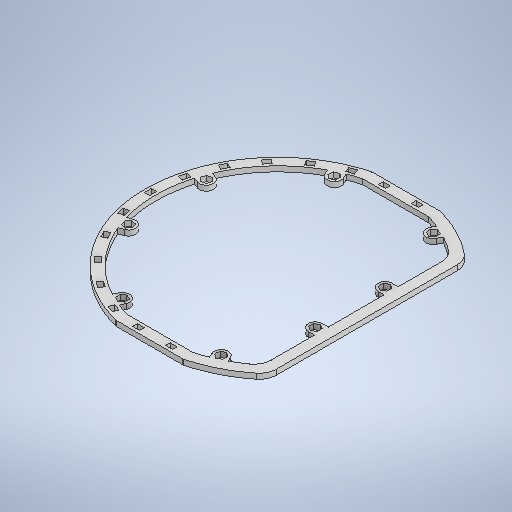
# Autodesk Inventor part: carcasa3.0
Saved by Autodesk Inventor 2025.3 (Build 293356030, 356C)
## iProperties
Created: 2025-08-27
Part Number: carcasa3.0
Material: Generic
Document SubType Name: Modeling
Designer: cdavi
Density: 1 g/cm^3
Appearance: Default
Author: cdavi
Autodesk Inventor part; units mm, degrees
ref_plane "YZ Plane" through (0, 0, 0) normal (1, 0, 0) x (0, 1, 0)
ref_plane "XZ Plane" through (0, 0, 0) normal (0, 1, 0) x (-1, 0, 0)
ref_plane "XY Plane" through (0, 0, 0) normal (0, 0, 1) x (1, 0, 0)
sketch "Sketch1" plane through (0, 0, 0) normal (0, 1, 0) x (-1, 0, 0)
  line L0 (18.2688, 67.5) -> (-18.2688, 67.5)
  line L1 (0, 0) -> (-51, 0) construction
  line L2 (19.0722, 73.5) -> (-19.0722, 73.5)
  line L3 (18.2688, -67.5) -> (-18.5405, -67.5)
  line L4 (19.0722, -73.5) -> (-19.0722, -73.5)
  line L5 (0, 0) -> (0, 73.5) construction
  line L6 (-45, 48.734) -> (-45, -48.734)
  line L7 (-51, 51.7204) -> (-51, -51.7204)
  arc A0 (-40.8333, -56.8563) -> (-18.5405, -67.5) centre (0, 0) ccw
  arc A1 (-47.2121, -59.5568) -> (-19.5877, -73.4324) centre (0, 0) ccw
  arc A2 (19.5877, -73.4324) -> (19.5877, 73.4324) centre (0, 0) ccw
  arc A3 (-19.5877, 73.4324) -> (-47.2121, 59.5568) centre (0, 0) ccw
  arc A4 (18.8061, -67.4265) -> (18.8061, 67.4265) centre (0, 0) ccw
  arc A5 (-18.8061, 67.4265) -> (-40.8333, 56.8563) centre (0, 0) ccw
  arc A6 (-19.5877, -73.4324) -> (-19.0722, -73.5) centre (-19.0722, -71.5) ccw
  arc A7 (19.0722, -73.5) -> (19.5877, -73.4324) centre (19.0722, -71.5) ccw
  arc A8 (18.2688, -67.5) -> (18.8061, -67.4265) centre (18.2688, -65.5) ccw
  arc A9 (18.8061, 67.4265) -> (18.2688, 67.5) centre (18.2688, 65.5) ccw
  arc A10 (19.5877, 73.4324) -> (19.0722, 73.5) centre (19.0722, 71.5) ccw
  arc A11 (-18.2688, 67.5) -> (-18.8061, 67.4265) centre (-18.2688, 65.5) ccw
  arc A12 (-19.0722, 73.5) -> (-19.5877, 73.4324) centre (-19.0722, 71.5) ccw
  arc A13 (-40.8333, 56.8563) -> (-45, 48.734) centre (-35, 48.734) ccw
  arc A14 (-47.2121, 59.5568) -> (-51, 51.7204) centre (-41, 51.7204) ccw
  arc A15 (-51, -51.7204) -> (-47.2121, -59.5568) centre (-41, -51.7204) ccw
  arc A16 (-45, -48.734) -> (-40.8333, -56.8563) centre (-35, -48.734) ccw
  point P0 (-19.3326, 73.5)
  point P1 (18.5405, -67.5)
  point P2 (19.3326, -73.5)
  point P3 (-19.3326, -73.5)
  point P4 (-51, -56.3471)
  point P5 (-45, 53.619)
  point P6 (-45, -53.619)
  point P7 (-51, 56.3471)
  point P8 (19.3326, 73.5)
  point P9 (18.5405, 67.5)
  point P10 (-18.5405, 67.5)
  dimension "d2" = 67.5
  dimension "d4" = 6
  dimension "d6" = 45
  dimension "d7" = 6
  dimension "d8" = 2
  dimension "d9" = 10
  dimension "d10" = 70
  dimension "d11" = 76
  dimension "d12" = 70
  dimension "d13" = 76
  constraints: 45 point on circle, 22 tangent, 17 centre point, 16 end point, 11 point on line, 9 equal radius, 4 symmetric about line, 3 vertical, 2 coincident, 2 horizontal, 2 midpoint, 1 parallel
  measures "d2" distance between parallel lines of L1 L0
  measures "d4" distance between parallel lines of L0 L2
  measures "d6" distance between parallel lines of L6 L5
  measures "d7" distance between parallel lines of L7 L6
  measures "d8" radius of A6
  measures "d9" radius of A13
  measures "d10" radius of A4
  measures "d11" radius of A2
  measures "d12" radius of A0
  measures "d13" radius of A1
extrude "Extrusion1" add sketch "Sketch1" along normal blind 65
sketch "Sketch2" plane through (51, 0, 51.7204) normal (1, 0, 0) x (0, 0, -1)
  line L0 (51.7204, 0) -> (51.7204, 65) construction
  line L1 (100.4544, 65) -> (2.9864, 65) projected
  line L2 (-2.712, 38) -> (17.288, 38)
  line L3 (17.288, 38) -> (17.288, 26)
  line L4 (17.288, 26) -> (-2.712, 26)
  line L5 (-2.712, 26) -> (-2.712, 38)
  line L6 (0, 0) -> (103.4408, 0) projected
  line L7 (-21.712, 0) -> (-21.712, 65) projected
  line L8 (106.1528, 38) -> (86.1528, 38)
  line L9 (86.1528, 38) -> (86.1528, 26)
  line L10 (86.1528, 26) -> (106.1528, 26)
  line L11 (106.1528, 26) -> (106.1528, 38)
  dimension "d16" = 26
  dimension "d17" = 19
  dimension "d18" = 12
  dimension "d19" = 20
  constraints: 18 end point, 4 symmetric about line, 2 parallel, 1 horizontal, 1 midpoint, 1 perpendicular
  measures "d16" distance between parallel lines of L6 L4
  measures "d17" distance between parallel lines of L5 L7
  measures "d18" distance of L2.end L3.end
  measures "d19" distance of L2.start L2.end
extrude "Extrusion2" cut sketch "Sketch2" against normal blind 5
sketch "Sketch3" plane through (51, 0, 51.7204) normal (1, 0, 0) x (0, 0, -1)
  line L0 (3.568, 49.2223) -> (17.7975, 43.9952) construction
  line L1 (2.8909, 47.379) -> (17.1204, 42.1519)
  line L2 (18.4746, 45.8385) -> (4.2452, 51.0656)
  arc A0 (4.2452, 51.0656) -> (2.8909, 47.379) centre (3.568, 49.2223) ccw
  arc A1 (17.1204, 42.1519) -> (18.4746, 45.8385) centre (17.7975, 43.9952) ccw
  arc A2 (44.4296, 11.624) -> (34.6921, 2.9774) centre (43.8866, 2.4292) ccw construction
  arc A3 (44.531, 13.3402) -> (32.9759, 3.0797) centre (43.8866, 2.4292) ccw
  arc A4 (44.3283, 9.9077) -> (36.4083, 2.8751) centre (43.8866, 2.4292) ccw
  arc A5 (44.3283, 9.9077) -> (44.531, 13.3402) centre (44.4296, 11.624) ccw
  arc A6 (32.9759, 3.0797) -> (36.4083, 2.8751) centre (34.6921, 2.9774) ccw
  line L3 (51.7204, 0) -> (51.7204, 65) construction
  line L4 (100.5499, 47.379) -> (86.3204, 42.1519)
  line L5 (84.9662, 45.8385) -> (99.1956, 51.0656)
  arc A7 (100.5499, 47.379) -> (99.1956, 51.0656) centre (99.8728, 49.2223) ccw
  arc A8 (84.9662, 45.8385) -> (86.3204, 42.1519) centre (85.6433, 43.9952) ccw
  point P0 (10.6828, 46.6088)
  constraints: 18 point on circle, 12 end point, 9 centre point, 8 tangent, 6 symmetric about line, 1 midpoint, 1 parallel, 2 other
extrude "Extrusion3" [suppressed]
extrude "Extrusion4" add sketch "Sketch1" along normal blind 3 from surface at 65 separate body contours A9 A4 A8 L3 A0 A16 L6 A13 A5 A11 L0 | A10 A2 A7 L4 A6 A1 A15 L7 A14 A3 A12 L2
sketch "Sketch5" plane through (-19.0722, 68, 73.5) normal (0, 1, 0) x (1, 0, 0)
  circle A0 centre (19.0722, 73.5) radius 8.5
  circle A1 centre (-10.9278, 73.5) radius 2.5
  line L0 (27.1963, 71) -> (36.0722, 71)
  line L1 (36.0722, 71) -> (36.0722, 76)
  line L2 (36.0722, 76) -> (27.1963, 76)
  point P0 (36.0722, 73.5)
  dimension "d26" = 17
  dimension "d27" = 5
  dimension "d31" = 5
  dimension "d32" = 17
  dimension "d47" = 30
  constraints: 6 end point, 2 centre point, 2 horizontal alignment, 2 perpendicular, 2 point on circle, 1 coincident, 1 horizontal, 1 midpoint
  measures "d26" diameter of A0
  measures "d27" diameter of A1
  measures "d31" distance between parallel lines of L2 L0
  measures "d32" distance from line of A0.centre L1
  measures "d47" distance of A0.centre A1.centre
extrude "Extrusion5" cut sketch "Sketch5" against normal through all bodies 2
sketch "Sketch6" plane through (0, 0, 0) normal (0, 1, 0) x (-1, 0, 0)
  circle A0 centre (0, 0) radius 67 construction
  arc A1 (-18.8061, 67.4265) -> (-40.8333, 56.8563) centre (0, 0) ccw projected
  arc A2 (-40.8333, 56.8563) -> (-45, 48.734) centre (-35, 48.734) ccw projected
  line L0 (-45, -48.734) -> (-45, 48.734) projected
  arc A3 (-45, -48.734) -> (-40.8333, -56.8563) centre (-35, -48.734) ccw projected
  arc A4 (-40.8333, -56.8563) -> (-18.5405, -67.5) centre (0, 0) ccw projected
  line L1 (18.2688, -67.5) -> (-18.5405, -67.5) construction
  arc A5 (18.8061, -67.4265) -> (18.8061, 67.4265) centre (0, 0) ccw projected
  line L2 (-18.2688, 67.5) -> (18.2688, 67.5) construction
  line L3 (19.0722, 73.5) -> (-19.0722, 73.5) projected
  arc A6 (-19.5877, 73.4324) -> (-47.2121, 59.5568) centre (0, 0) ccw projected
  arc A7 (-47.2121, 59.5568) -> (-51, 51.7204) centre (-41, 51.7204) ccw projected
  line L4 (-51, 51.7204) -> (-51, -51.7204) projected
  arc A8 (-51, -51.7204) -> (-47.2121, -59.5568) centre (-41, -51.7204) ccw projected
  arc A9 (-47.2121, -59.5568) -> (-19.5877, -73.4324) centre (0, 0) ccw projected
  line L5 (-19.0722, -73.5) -> (19.0722, -73.5) projected
  arc A10 (19.5877, -73.4324) -> (19.5877, 73.4324) centre (0, 0) ccw projected
  arc A11 (-17.9906, 61.4194) -> (-37.3333, 51.9829) centre (0, 0) ccw construction
  arc A12 (-37.3333, 51.9829) -> (-39, 48.734) centre (-35, 48.734) ccw construction
  line L6 (-39, 48.734) -> (-39, -48.734) construction
  arc A13 (-39, -48.734) -> (-37.3333, -51.9829) centre (-35, -48.734) ccw construction
  arc A14 (-37.3333, -51.9829) -> (-17.9906, -61.4194) centre (0, 0) ccw construction
  line L7 (-17.4284, -61.5) -> (17.4284, -61.5) construction
  line L8 (-17.4284, 61.5) -> (17.4284, 61.5) construction
  arc A15 (17.9906, -61.4194) -> (17.9906, 61.4194) centre (0, 0) ccw construction
  arc A16 (-8.124, -2.5) -> (-8.124, 2.5) centre (0, 0) ccw projected
  line L9 (0, 0) -> (63.1919, 22.2662) construction
  line L10 (0, 0) -> (76, 0) construction
  circle A17 centre (63.1919, 22.2662) radius 2.85 construction
  line L11 (0, 0) -> (0, -67) construction
  circle A18 centre (28.3154, 60.7226) radius 2.85 construction
  line L12 (28.3154, 60.7226) -> (0, 0) construction
  circle A19 centre (-41.5, 20) radius 2.85 construction
  circle A20 centre (-28.3154, 60.7226) radius 2.85 construction
  line L13 (-28.3154, 60.7226) -> (0, 0) construction
  arc A21 (-17.4284, 61.5) -> (-17.9906, 61.4194) centre (-17.4284, 59.5) ccw construction
  arc A22 (-17.9906, -61.4194) -> (-17.4284, -61.5) centre (-17.4284, -59.5) ccw construction
  arc A23 (17.4284, -61.5) -> (17.9906, -61.4194) centre (17.4284, -59.5) ccw construction
  arc A24 (17.9906, 61.4194) -> (17.4284, 61.5) centre (17.4284, 59.5) ccw construction
  arc A25 (-19.5877, -73.4324) -> (-19.0722, -73.5) centre (-19.0722, -71.5) ccw projected
  arc A26 (19.0722, -73.5) -> (19.5877, -73.4324) centre (19.0722, -71.5) ccw projected
  arc A27 (19.5877, 73.4324) -> (19.0722, 73.5) centre (19.0722, 71.5) ccw projected
  arc A28 (-19.0722, 73.5) -> (-19.5877, 73.4324) centre (-19.0722, 71.5) ccw projected
  circle A29 centre (63.1919, -22.2662) radius 2.85 construction
  circle A30 centre (28.3154, -60.7226) radius 2.85 construction
  circle A31 centre (-41.5, -20) radius 2.85 construction
  circle A32 centre (-28.3154, -60.7226) radius 2.85 construction
  line L14 (18.8061, 61.1746) -> (18.8061, 67.4265)
  line L15 (-18.8061, 61.1746) -> (-18.8061, 67.4265)
  line L16 (18.8061, 67.4265) -> (-18.8061, 67.4265)
  line L17 (18.8061, -61.1746) -> (18.8061, -67.4265)
  line L18 (-18.8061, -61.1746) -> (-18.8061, -67.4265)
  line L19 (18.8061, -67.4265) -> (-18.8061, -67.4265)
  circle A33 centre (63.1919, 22.2662) radius 4
  circle A34 centre (28.3154, 60.7226) radius 4
  line L20 (60.3905, 22.7899) -> (62.2448, 24.9542)
  line L21 (62.2448, 24.9542) -> (65.0462, 24.4304)
  line L22 (65.0462, 24.4304) -> (65.9934, 21.7424)
  line L23 (65.9934, 21.7424) -> (64.1391, 19.5782)
  line L24 (64.1391, 19.5782) -> (61.3376, 20.1019)
  line L25 (61.3376, 20.1019) -> (60.3905, 22.7899)
  line L26 (25.9808, 59.0879) -> (25.7324, 61.9271)
  line L27 (25.7324, 61.9271) -> (28.067, 63.5618)
  line L28 (28.067, 63.5618) -> (30.65, 62.3573)
  line L29 (30.65, 62.3573) -> (30.8984, 59.5182)
  line L30 (30.8984, 59.5182) -> (28.5638, 57.8835)
  line L31 (28.5638, 57.8835) -> (25.9808, 59.0879)
  circle A35 centre (-41.5, 20) radius 4
  line L32 (-43.9682, 18.575) -> (-43.9682, 21.425)
  line L33 (-43.9682, 21.425) -> (-41.5, 22.85)
  line L34 (-41.5, 22.85) -> (-39.0318, 21.425)
  line L35 (-39.0318, 21.425) -> (-39.0318, 18.575)
  line L36 (-39.0318, 18.575) -> (-41.5, 17.15)
  line L37 (-41.5, 17.15) -> (-43.9682, 18.575)
  line L38 (-41.5, 24) -> (-45, 24)
  line L39 (-41.5, 16) -> (-45, 16)
  circle A36 centre (-28.3154, 60.7226) radius 4
  line L40 (-28.5638, 57.8835) -> (-30.8984, 59.5182)
  line L41 (-30.8984, 59.5182) -> (-30.65, 62.3573)
  line L42 (-30.65, 62.3573) -> (-28.067, 63.5618)
  line L43 (-28.067, 63.5618) -> (-25.7324, 61.9271)
  line L44 (-25.7324, 61.9271) -> (-25.9808, 59.0879)
  line L45 (-25.9808, 59.0879) -> (-28.5638, 57.8835)
  line L46 (-31.8886, 58.9247) -> (-33.2376, 61.6057)
  circle A37 centre (63.1919, -22.2662) radius 4
  circle A38 centre (28.3154, -60.7226) radius 4
  circle A39 centre (-41.5, -20) radius 4
  line L47 (-41.5, -24) -> (-45, -24)
  line L48 (-41.5, -16) -> (-45, -16)
  circle A40 centre (-28.3154, -60.7226) radius 4
  line L49 (-31.8886, -58.9247) -> (-33.2376, -61.6057)
  line L50 (60.3905, -22.7899) -> (62.2448, -24.9542)
  line L51 (62.2448, -24.9542) -> (65.0462, -24.4304)
  line L52 (65.0462, -24.4304) -> (65.9934, -21.7424)
  line L53 (65.9934, -21.7424) -> (64.1391, -19.5782)
  line L54 (64.1391, -19.5782) -> (61.3376, -20.1019)
  line L55 (61.3376, -20.1019) -> (60.3905, -22.7899)
  line L56 (25.9808, -59.0879) -> (25.7324, -61.9271)
  line L57 (25.7324, -61.9271) -> (28.067, -63.5618)
  line L58 (28.067, -63.5618) -> (30.65, -62.3573)
  line L59 (30.65, -62.3573) -> (30.8984, -59.5182)
  line L60 (30.8984, -59.5182) -> (28.5638, -57.8835)
  line L61 (28.5638, -57.8835) -> (25.9808, -59.0879)
  line L62 (-28.5638, -57.8835) -> (-30.8984, -59.5182)
  line L63 (-30.8984, -59.5182) -> (-30.65, -62.3573)
  line L64 (-30.65, -62.3573) -> (-28.067, -63.5618)
  line L65 (-28.067, -63.5618) -> (-25.7324, -61.9271)
  line L66 (-25.7324, -61.9271) -> (-25.9808, -59.0879)
  line L67 (-25.9808, -59.0879) -> (-28.5638, -57.8835)
  line L68 (-43.9682, -18.575) -> (-43.9682, -21.425)
  line L69 (-43.9682, -21.425) -> (-41.5, -22.85)
  line L70 (-41.5, -22.85) -> (-39.0318, -21.425)
  line L71 (-39.0318, -21.425) -> (-39.0318, -18.575)
  line L72 (-39.0318, -18.575) -> (-41.5, -17.15)
  line L73 (-41.5, -17.15) -> (-43.9682, -18.575)
  line L74 (61.7506, 25.9975) -> (64.5502, 27.0789)
  line L75 (64.408, 18.4555) -> (67.2672, 19.368)
  line L76 (31.8886, 58.9247) -> (33.2376, 61.6057)
  line L77 (61.7506, -25.9975) -> (64.5502, -27.0789)
  line L78 (64.408, -18.4555) -> (67.2672, -19.368)
  line L79 (31.8886, -58.9247) -> (33.2376, -61.6057)
  line L80 (-24.6413, 62.3041) -> (-25.828, 65.0609)
  line L81 (24.6413, 62.3041) -> (25.828, 65.0609)
  line L82 (-24.6413, -62.3041) -> (-25.828, -65.0609)
  line L83 (24.6413, -62.3041) -> (25.828, -65.0609)
  point P0 (-17.713, -61.5)
  point P1 (-18.8061, 61.1746)
  point P2 (18.8061, -61.1746)
  point P3 (-18.8061, -61.1746)
  point P4 (28.3154, 60.7226)
  point P5 (28.3154, 60.7226)
  point P6 (-18.8061, -67.4265)
  point P7 (-27.1107, 64.5369)
  point P8 (-27.1107, -64.5369)
  point P9 (27.1107, -64.5369)
  point P10 (27.1107, 64.5369)
  point P11 (-45, 21.9365)
  point P12 (-45, 18.0635)
  point P13 (-32.0117, 62.2515)
  point P14 (32.0117, -62.2515)
  point P15 (66.8707, -20.6956)
  point P16 (65.0736, -25.796)
  point P17 (-32.0117, -62.2515)
  point P18 (-45, -21.9365)
  point P19 (-45, -18.0635)
  point P20 (65.0736, 25.796)
  point P21 (66.8707, 20.6956)
  point P22 (32.0117, 62.2515)
  dimension "d33" = 134
  dimension "d39" = 5.7
  dimension "d34" = 6
  dimension "d35" = 6
  dimension "d36" = 6
  dimension "d37" = 19.41
  dimension "d38" = 25
  dimension "d40" = 20
  dimension "d41" = 3.5
  dimension "d42" = 25
  dimension "d44" = 2
  dimension "d61" = 8
  dimension "d62" = 8
  dimension "d63" = 8
  dimension "d64" = 8
  constraints: 156 end point, 52 symmetric about line, 37 point on circle, 20 centre point, 16 tangent, 10 coincident, 6 perpendicular, 3 equal radius, 3 point on line, 2 parallel, 2 vertical, 93 other
  measures "d34" radial gap between concentric circles of A1 A11
  measures "d35" distance between parallel lines of L2 L8
  measures "d36" radial gap between concentric circles of A5 A15
  measures "d37" angle of L10 L9
  measures "d38" angle of L11 L12
  measures "d40" distance from line of point (-41.5, 20) L10
  measures "d41" distance from line of L0 point (-41.5, 20)
  measures "d42" angle of L11 L13
  measures "d44" radius of A21
  measures "d61" diameter of A33
  measures "d62" diameter of A34
  measures "d63" diameter of A35
  measures "d64" diameter of A36
extrude "Extrusion6" add sketch "Sketch6" against normal blind 3 separate body contours L80 A36 A1 | A36 A1 | A1 A36 | A5 A34 L81 | A36 L46 A1 | A34 A5 | A5 A34 | A5 L76 A34 | A5 A33 L74 | L38 A35 L0 | A33 A5 | A5 A33 | A35 L0 | L0 A35 | A5 L75 A33 | A35 L39 L0 | A5 A37 L78 | L48 A39 L0 | A37 A5 | A5 A37 | A39 L0 | L0 A39 | A5 L77 A37 | A39 L47 L0 | A5 A38 L79 | A38 A5 | A5 A38 | A5 L83 A38 | L49 A40 A4 | A40 A4 | A4 A40 | A40 L82 A4 | A27 A10 A26 L5 A25 A9 A8 L4 A7 A6 A28 L3
sketch "Sketch7" plane through (0, 0, 0) normal (0, 1, 0) x (1, 0, 0)
  line L0 (-43.1612, -69.503) -> (-43.1612, 69.6172)
  line L1 (-23.8326, -59.397) -> (-23.8326, -67.4265) projected
  line L2 (-94.0019, 0.3288) -> (-72.5423, 0.3288)
  line L3 (-72.5423, 0.3288) -> (-72.5423, -7.6712)
  line L4 (-72.5423, 0.3288) -> (-72.5423, 8.3288)
  arc A0 (-19.5877, 73.4324) -> (-19.5877, -73.4324) centre (0, 0) ccw projected
  line L5 (-72.5423, -7.6712) -> (-75.5423, -7.6712)
  line L6 (-75.5423, -7.6712) -> (-75.5423, 8.3288)
  line L7 (-75.5423, 8.3288) -> (-72.5423, 8.3288)
  line L8 (-68.8178, -24.1938) -> (-71.7369, -24.8857)
  line L9 (-71.7369, -24.8857) -> (-75.4267, -9.317)
  line L10 (-70.6627, -16.4095) -> (-68.8178, -24.1938)
  line L11 (-70.6627, -16.4095) -> (-72.5076, -8.6251)
  line L12 (-75.4267, -9.317) -> (-72.5076, -8.6251)
  line L13 (-61.3833, -39.4122) -> (-64.0642, -40.7586)
  line L14 (-64.0642, -40.7586) -> (-71.245, -26.4604)
  line L15 (-64.9737, -32.2631) -> (-61.3833, -39.4122)
  line L16 (-64.9737, -32.2631) -> (-68.5641, -25.114)
  line L17 (-71.245, -26.4604) -> (-68.5641, -25.114)
  line L18 (-50.6396, -52.5058) -> (-52.9377, -54.4341)
  line L19 (-52.9377, -54.4341) -> (-63.2223, -42.1774)
  line L20 (-55.7819, -46.3774) -> (-50.6396, -52.5058)
  line L21 (-55.7819, -46.3774) -> (-60.9242, -40.2491)
  line L22 (-63.2223, -42.1774) -> (-60.9242, -40.2491)
  line L23 (-37.166, -62.7688) -> (-38.9574, -65.1751)
  line L24 (-38.9574, -65.1751) -> (-51.7914, -55.6206)
  line L25 (-43.5829, -57.9915) -> (-37.166, -62.7688)
  line L26 (-43.5829, -57.9915) -> (-49.9999, -53.2142)
  line L27 (-51.7914, -55.6206) -> (-49.9999, -53.2142)
  line L28 (-21.6887, -69.6479) -> (-22.8769, -72.4025)
  line L29 (-22.8769, -72.4025) -> (-37.5684, -66.0653)
  line L30 (-29.0344, -66.4792) -> (-21.6887, -69.6479)
  line L31 (-29.0344, -66.4792) -> (-36.3801, -63.3106)
  line L32 (-37.5684, -66.0653) -> (-36.3801, -63.3106)
  line L33 (-5.0421, -72.7723) -> (-5.5631, -75.7267)
  line L34 (-5.5631, -75.7267) -> (-21.32, -72.9483)
  line L35 (-12.9206, -71.3831) -> (-5.0421, -72.7723)
  line L36 (-12.9206, -71.3831) -> (-20.7991, -69.9939)
  line L37 (-21.32, -72.9483) -> (-20.7991, -69.9939)
  line L38 (11.8762, -71.9735) -> (12.0506, -74.9684)
  line L39 (12.0506, -74.9684) -> (-3.9223, -75.8987)
  line L40 (3.8897, -72.4386) -> (11.8762, -71.9735)
  line L41 (3.8897, -72.4386) -> (-4.0967, -72.9038)
  line L42 (-3.9223, -75.8987) -> (-4.0967, -72.9038)
  line L43 (28.1543, -67.2946) -> (29.0147, -70.1685)
  line L44 (29.0147, -70.1685) -> (13.6869, -74.7574)
  line L45 (20.4904, -69.589) -> (28.1543, -67.2946)
  line L46 (20.4904, -69.589) -> (12.8265, -71.8834)
  line L47 (13.6869, -74.7574) -> (12.8265, -71.8834)
  line L48 (42.9146, -58.9878) -> (44.4146, -61.5859)
  line L49 (44.4146, -61.5859) -> (30.5582, -69.5859)
  line L50 (35.9864, -62.9878) -> (42.9146, -58.9878)
  line L51 (35.9864, -62.9878) -> (29.0582, -66.9878)
  line L52 (30.5582, -69.5859) -> (29.0582, -66.9878)
  line L53 (55.3614, -47.501) -> (57.4201, -49.6831)
  line L54 (57.4201, -49.6831) -> (45.7821, -60.663)
  line L55 (49.5424, -52.9909) -> (55.3614, -47.501)
  line L56 (49.5424, -52.9909) -> (43.7234, -58.4809)
  line L57 (45.7821, -60.663) -> (43.7234, -58.4809)
  line L58 (64.8236, -33.4534) -> (67.33, -35.1019)
  line L59 (67.33, -35.1019) -> (58.5379, -48.4697)
  line L60 (60.4275, -40.1373) -> (64.8236, -33.4534)
  line L61 (60.4275, -40.1373) -> (56.0314, -46.8212)
  line L62 (58.5379, -48.4697) -> (56.0314, -46.8212)
  line L63 (70.7911, -17.6023) -> (73.6102, -18.6284)
  line L64 (73.6102, -18.6284) -> (68.1379, -33.6635)
  line L65 (68.055, -25.1199) -> (70.7911, -17.6023)
  line L66 (68.055, -25.1199) -> (65.3188, -32.6374)
  line L67 (68.1379, -33.6635) -> (65.3188, -32.6374)
  line L68 (72.9423, -0.8023) -> (75.922, -1.1506)
  line L69 (75.922, -1.1506) -> (74.0646, -17.0424)
  line L70 (72.0136, -8.7482) -> (72.9423, -0.8023)
  line L71 (72.0136, -8.7482) -> (71.0848, -16.6941)
  line L72 (74.0646, -17.0424) -> (71.0848, -16.6941)
  line L73 (71.1612, 16.041) -> (74.1409, 16.3893)
  line L74 (74.1409, 16.3893) -> (75.9984, 0.4975)
  line L75 (72.0899, 8.0951) -> (71.1612, 16.041)
  line L76 (72.0899, 8.0951) -> (73.0187, 0.1492)
  line L77 (75.9984, 0.4975) -> (73.0187, 0.1492)
  line L78 (65.5437, 32.0195) -> (68.3628, 33.0456)
  line L79 (68.3628, 33.0456) -> (73.8351, 18.0105)
  line L80 (68.2799, 24.502) -> (65.5437, 32.0195)
  line L81 (68.2799, 24.502) -> (71.016, 16.9844)
  line L82 (73.8351, 18.0105) -> (71.016, 16.9844)
  line L83 (56.3928, 46.2718) -> (58.8992, 47.9204)
  line L84 (58.8992, 47.9204) -> (67.6914, 34.5526)
  line L85 (60.7888, 39.5879) -> (56.3928, 46.2718)
  line L86 (60.7888, 39.5879) -> (65.1849, 32.904)
  line L87 (67.6914, 34.5526) -> (65.1849, 32.904)
  line L88 (44.2017, 58.0296) -> (46.2604, 60.2118)
  line L89 (46.2604, 60.2118) -> (57.8984, 49.2319)
  line L90 (50.0206, 52.5397) -> (44.2017, 58.0296)
  line L91 (50.0206, 52.5397) -> (55.8396, 47.0498)
  line L92 (57.8984, 49.2319) -> (55.8396, 47.0498)
  line L93 (29.6276, 66.659) -> (31.1276, 69.2571)
  line L94 (31.1276, 69.2571) -> (44.984, 61.2571)
  line L95 (36.5558, 62.659) -> (29.6276, 66.659)
  line L96 (36.5558, 62.659) -> (43.484, 58.659)
  line L97 (44.984, 61.2571) -> (43.484, 58.659)
  line L98 (13.4564, 71.6948) -> (14.3168, 74.5688)
  line L99 (14.3168, 74.5688) -> (29.6446, 69.98)
  line L100 (21.1203, 69.4004) -> (13.4564, 71.6948)
  line L101 (21.1203, 69.4004) -> (28.7842, 67.106)
  line L102 (29.6446, 69.98) -> (28.7842, 67.106)
  line L103 (-3.4403, 72.8656) -> (-3.2659, 75.8605)
  line L104 (-3.2659, 75.8605) -> (12.7071, 74.9302)
  line L105 (4.5462, 72.4004) -> (-3.4403, 72.8656)
  line L106 (4.5462, 72.4004) -> (12.5326, 71.9352)
  line L107 (12.7071, 74.9302) -> (12.5326, 71.9352)
  line L108 (-20.1515, 70.1081) -> (-20.6725, 73.0625)
  line L109 (-20.6725, 73.0625) -> (-4.9155, 75.8409)
  line L110 (-12.2731, 71.4973) -> (-20.1515, 70.1081)
  line L111 (-12.2731, 71.4973) -> (-4.3946, 72.8864)
  line L112 (-4.9155, 75.8409) -> (-4.3946, 72.8864)
  line L113 (-35.7764, 63.571) -> (-36.9646, 66.3257)
  line L114 (-36.9646, 66.3257) -> (-22.2731, 72.663)
  line L115 (-28.4306, 66.7397) -> (-35.7764, 63.571)
  line L116 (-28.4306, 66.7397) -> (-21.0849, 69.9083)
  line L117 (-22.2731, 72.663) -> (-21.0849, 69.9083)
  line L118 (-49.4725, 53.6069) -> (-51.264, 56.0132)
  line L119 (-51.264, 56.0132) -> (-38.43, 65.5678)
  line L120 (-43.0555, 58.3841) -> (-49.4725, 53.6069)
  line L121 (-43.0555, 58.3841) -> (-36.6385, 63.1614)
  line L122 (-38.43, 65.5678) -> (-36.6385, 63.1614)
  line L123 (-60.5016, 40.7528) -> (-62.7997, 42.6811)
  line L124 (-62.7997, 42.6811) -> (-52.5151, 54.9378)
  line L125 (-55.3593, 46.8811) -> (-60.5016, 40.7528)
  line L126 (-55.3593, 46.8811) -> (-50.217, 53.0095)
  line L127 (-52.5151, 54.9378) -> (-50.217, 53.0095)
  line L128 (-68.269, 25.7016) -> (-70.9499, 27.048)
  line L129 (-70.9499, 27.048) -> (-63.7691, 41.3462)
  line L130 (-64.6786, 32.8507) -> (-68.269, 25.7016)
  line L131 (-64.6786, 32.8507) -> (-61.0882, 39.9998)
  line L132 (-63.7691, 41.3462) -> (-61.0882, 39.9998)
  line L133 (-72.356, 9.2649) -> (-75.2751, 9.9568)
  line L134 (-75.2751, 9.9568) -> (-71.5853, 25.5255)
  line L135 (-70.511, 17.0493) -> (-72.356, 9.2649)
  line L136 (-70.511, 17.0493) -> (-68.6661, 24.8337)
  line L137 (-71.5853, 25.5255) -> (-68.6661, 24.8337)
  line L138 (-43.1612, 0.3288) -> (-94.0019, 0.3288)
  arc A1 (-43.1612, 55.2979) -> (-23.8326, -59.397) centre (-20.9962, 0.0571) ccw
  arc A2 (-20.6725, 73.0625) -> (-21.32, -72.9483) centre (-20.9962, 0.0571) ccw
  point P0 (-43.1612, -69.503)
  point P1 (-18.8061, -67.4265)
  dimension "d49" = 8
  dimension "d51" = 3
  dimension "d52" = 16
  dimension "d55" = 360
  constraints: 275 end point, 7 point on circle, 2 centre point, 2 perpendicular, 1 coincident, 1 horizontal, 1 point on line, 1 vertical, 278 other
  measures "d49" distance of L2.end L3.end
  measures "d51" distance of L3.end L5.end
  measures "d52" distance of L5.end L6.end
sketch "Sketch8" plane through (0, 0, 0) normal (0, 1, 0) x (1, 0, 0)
  arc A0 (-19.5877, 73.4324) -> (-19.5877, -73.4324) centre (0, 0) ccw projected
  line L0 (-76, 0) -> (-70, 0)
  arc A1 (-67.2672, 19.368) -> (-67.2672, -19.368) centre (0, 0) ccw projected
  line L1 (-73, 0) -> (-73, -2)
  line L2 (-73, 0) -> (-73, 2)
  line L3 (-73, 2) -> (-71.5, 2)
  line L4 (-71.5, 2) -> (-71.5, -2)
  line L5 (-71.5, -2) -> (-74.5, -2)
  line L6 (-74.5, -2) -> (-74.5, 2)
  line L7 (-74.5, 2) -> (-71.5, 2)
  line L8 (-69.901, -15.1692) -> (-68.9437, -19.053)
  line L9 (-68.9437, -19.053) -> (-71.8565, -19.7709)
  line L10 (-71.8565, -19.7709) -> (-72.8138, -15.8871)
  line L11 (-71.3574, -15.5282) -> (-69.901, -15.1692)
  line L12 (-72.8138, -15.8871) -> (-69.901, -15.1692)
  line L13 (-64.2396, -31.4568) -> (-62.3807, -34.9986)
  line L14 (-62.3807, -34.9986) -> (-65.037, -36.3928)
  line L15 (-65.037, -36.3928) -> (-66.8959, -32.851)
  line L16 (-65.5677, -32.1539) -> (-64.2396, -31.4568)
  line L17 (-66.8959, -32.851) -> (-64.2396, -31.4568)
  line L18 (-54.8448, -45.9162) -> (-52.1923, -48.9103)
  line L19 (-52.1923, -48.9103) -> (-54.4378, -50.8997)
  line L20 (-54.4378, -50.8997) -> (-57.0903, -47.9056)
  line L21 (-55.9675, -46.9109) -> (-54.8448, -45.9162)
  line L22 (-57.0903, -47.9056) -> (-54.8448, -45.9162)
  line L23 (-42.2626, -57.7072) -> (-38.9707, -59.9795)
  line L24 (-38.9707, -59.9795) -> (-40.6749, -62.4484)
  line L25 (-40.6749, -62.4484) -> (-43.9668, -60.1762)
  line L26 (-43.1147, -58.9417) -> (-42.2626, -57.7072)
  line L27 (-43.9668, -60.1762) -> (-42.2626, -57.7072)
  line L28 (-27.2243, -66.1445) -> (-23.4842, -67.5629)
  line L29 (-23.4842, -67.5629) -> (-24.548, -70.3679)
  line L30 (-24.548, -70.3679) -> (-28.2881, -68.9495)
  line L31 (-27.7562, -67.547) -> (-27.2243, -66.1445)
  line L32 (-28.2881, -68.9495) -> (-27.2243, -66.1445)
  line L33 (-10.6038, -70.7376) -> (-6.633, -71.2198)
  line L34 (-6.633, -71.2198) -> (-6.9946, -74.1979)
  line L35 (-6.9946, -74.1979) -> (-10.9654, -73.7157)
  line L36 (-10.7846, -72.2267) -> (-10.6038, -70.7376)
  line L37 (-10.9654, -73.7157) -> (-10.6038, -70.7376)
  line L38 (6.633, -71.2198) -> (10.6038, -70.7376)
  line L39 (10.6038, -70.7376) -> (10.9654, -73.7157)
  line L40 (10.9654, -73.7157) -> (6.9946, -74.1979)
  line L41 (6.8138, -72.7088) -> (6.633, -71.2198)
  line L42 (6.9946, -74.1979) -> (6.633, -71.2198)
  line L43 (23.4842, -67.5629) -> (27.2243, -66.1445)
  line L44 (27.2243, -66.1445) -> (28.2881, -68.9495)
  line L45 (28.2881, -68.9495) -> (24.548, -70.3679)
  line L46 (24.0161, -68.9654) -> (23.4842, -67.5629)
  line L47 (24.548, -70.3679) -> (23.4842, -67.5629)
  line L48 (38.9707, -59.9795) -> (42.2626, -57.7072)
  line L49 (42.2626, -57.7072) -> (43.9668, -60.1762)
  line L50 (43.9668, -60.1762) -> (40.6749, -62.4484)
  line L51 (39.8228, -61.214) -> (38.9707, -59.9795)
  line L52 (40.6749, -62.4484) -> (38.9707, -59.9795)
  line L53 (52.1923, -48.9103) -> (54.8448, -45.9162)
  line L54 (54.8448, -45.9162) -> (57.0903, -47.9056)
  line L55 (57.0903, -47.9056) -> (54.4378, -50.8997)
  line L56 (53.315, -49.905) -> (52.1923, -48.9103)
  line L57 (54.4378, -50.8997) -> (52.1923, -48.9103)
  line L58 (62.3807, -34.9986) -> (64.2396, -31.4568)
  line L59 (64.2396, -31.4568) -> (66.8959, -32.851)
  line L60 (66.8959, -32.851) -> (65.037, -36.3928)
  line L61 (63.7088, -35.6957) -> (62.3807, -34.9986)
  line L62 (65.037, -36.3928) -> (62.3807, -34.9986)
  line L63 (68.9437, -19.053) -> (69.901, -15.1692)
  line L64 (69.901, -15.1692) -> (72.8138, -15.8871)
  line L65 (72.8138, -15.8871) -> (71.8565, -19.7709)
  line L66 (70.4001, -19.4119) -> (68.9437, -19.053)
  line L67 (71.8565, -19.7709) -> (68.9437, -19.053)
  line L68 (71.5, -2) -> (71.5, 2)
  line L69 (71.5, 2) -> (74.5, 2)
  line L70 (74.5, 2) -> (74.5, -2)
  line L71 (73, -2) -> (71.5, -2)
  line L72 (74.5, -2) -> (71.5, -2)
  line L73 (69.901, 15.1692) -> (68.9437, 19.053)
  line L74 (68.9437, 19.053) -> (71.8565, 19.7709)
  line L75 (71.8565, 19.7709) -> (72.8138, 15.8871)
  line L76 (71.3574, 15.5282) -> (69.901, 15.1692)
  line L77 (72.8138, 15.8871) -> (69.901, 15.1692)
  line L78 (64.2396, 31.4568) -> (62.3807, 34.9986)
  line L79 (62.3807, 34.9986) -> (65.037, 36.3928)
  line L80 (65.037, 36.3928) -> (66.8959, 32.851)
  line L81 (65.5677, 32.1539) -> (64.2396, 31.4568)
  line L82 (66.8959, 32.851) -> (64.2396, 31.4568)
  line L83 (54.8448, 45.9162) -> (52.1923, 48.9103)
  line L84 (52.1923, 48.9103) -> (54.4378, 50.8997)
  line L85 (54.4378, 50.8997) -> (57.0903, 47.9056)
  line L86 (55.9675, 46.9109) -> (54.8448, 45.9162)
  line L87 (57.0903, 47.9056) -> (54.8448, 45.9162)
  line L88 (42.2626, 57.7072) -> (38.9707, 59.9795)
  line L89 (38.9707, 59.9795) -> (40.6749, 62.4484)
  line L90 (40.6749, 62.4484) -> (43.9668, 60.1762)
  line L91 (43.1147, 58.9417) -> (42.2626, 57.7072)
  line L92 (43.9668, 60.1762) -> (42.2626, 57.7072)
  line L93 (27.2243, 66.1445) -> (23.4842, 67.5629)
  line L94 (23.4842, 67.5629) -> (24.548, 70.3679)
  line L95 (24.548, 70.3679) -> (28.2881, 68.9495)
  line L96 (27.7562, 67.547) -> (27.2243, 66.1445)
  line L97 (28.2881, 68.9495) -> (27.2243, 66.1445)
  line L98 (10.6038, 70.7376) -> (6.633, 71.2198)
  line L99 (6.633, 71.2198) -> (6.9946, 74.1979)
  line L100 (6.9946, 74.1979) -> (10.9654, 73.7157)
  line L101 (10.7846, 72.2267) -> (10.6038, 70.7376)
  line L102 (10.9654, 73.7157) -> (10.6038, 70.7376)
  line L103 (-6.633, 71.2198) -> (-10.6038, 70.7376)
  line L104 (-10.6038, 70.7376) -> (-10.9654, 73.7157)
  line L105 (-10.9654, 73.7157) -> (-6.9946, 74.1979)
  line L106 (-6.8138, 72.7088) -> (-6.633, 71.2198)
  line L107 (-6.9946, 74.1979) -> (-6.633, 71.2198)
  line L108 (-23.4842, 67.5629) -> (-27.2243, 66.1445)
  line L109 (-27.2243, 66.1445) -> (-28.2881, 68.9495)
  line L110 (-28.2881, 68.9495) -> (-24.548, 70.3679)
  line L111 (-24.0161, 68.9654) -> (-23.4842, 67.5629)
  line L112 (-24.548, 70.3679) -> (-23.4842, 67.5629)
  line L113 (-38.9707, 59.9795) -> (-42.2626, 57.7072)
  line L114 (-42.2626, 57.7072) -> (-43.9668, 60.1762)
  line L115 (-43.9668, 60.1762) -> (-40.6749, 62.4484)
  line L116 (-39.8228, 61.214) -> (-38.9707, 59.9795)
  line L117 (-40.6749, 62.4484) -> (-38.9707, 59.9795)
  line L118 (-52.1923, 48.9103) -> (-54.8448, 45.9162)
  line L119 (-54.8448, 45.9162) -> (-57.0903, 47.9056)
  line L120 (-57.0903, 47.9056) -> (-54.4378, 50.8997)
  line L121 (-53.315, 49.905) -> (-52.1923, 48.9103)
  line L122 (-54.4378, 50.8997) -> (-52.1923, 48.9103)
  line L123 (-62.3807, 34.9986) -> (-64.2396, 31.4568)
  line L124 (-64.2396, 31.4568) -> (-66.8959, 32.851)
  line L125 (-66.8959, 32.851) -> (-65.037, 36.3928)
  line L126 (-63.7088, 35.6957) -> (-62.3807, 34.9986)
  line L127 (-65.037, 36.3928) -> (-62.3807, 34.9986)
  line L128 (-68.9437, 19.053) -> (-69.901, 15.1692)
  line L129 (-69.901, 15.1692) -> (-72.8138, 15.8871)
  line L130 (-72.8138, 15.8871) -> (-71.8565, 19.7709)
  line L131 (-70.4001, 19.4119) -> (-68.9437, 19.053)
  line L132 (-71.8565, 19.7709) -> (-68.9437, 19.053)
  dimension "d132" = 2
  dimension "d133" = 2
  dimension "d134" = 1.5
  dimension "d135" = 4
  dimension "d136" = 3
  dimension "d137" = 4
  dimension "d140" = 360
  constraints: 266 end point, 26 point on line, 3 perpendicular, 2 point on circle, 2 vertical, 1 horizontal, 1 midpoint, 261 other
  measures "d132" distance of L1.start L1.end
  measures "d133" distance of L1.start L2.end
  measures "d134" distance of L2.end L3.end
  measures "d135" distance of L3.end L4.end
  measures "d136" distance of L4.end L5.end
  measures "d137" distance of L5.end L6.end
extrude "Extrusion7" cut sketch "Sketch8" against normal blind 20.75 contours L6 L7 L2 L0 | L0 L1 L5 L6 | L2 L3 L4 L0 | L0 L4 L5 L1 | L8 L9 L10 L12 L11 | L13 L14 L15 L17 L16 | L18 L19 L20 L22 L21 | L23 L24 L25 L27 L26 | L28 L29 L30 L32 L31 | L108 L109 L110 L112 L111 | L113 L114 L115 L117 L116 | L118 L119 L120 L122 L121 | L123 L124 L125 L127 L126 | L128 L129 L130 L132 L131 bodies 3
sketch "Sketch9" plane through (0, 0, 0) normal (0, 1, 0) x (1, 0, 0)
  line L0 (18.8061, -67.4265) -> (-18.8061, -67.4265) projected
  line L1 (19.0722, -73.5) -> (-19.0722, -73.5) projected
  line L2 (-18.8061, -67.4265) -> (-18.8061, -73.5)
  line L3 (18.8061, -67.4265) -> (18.8061, -73.5)
  line L4 (-18.8061, -70.4632) -> (18.8061, -70.4632)
  line L5 (0, -70.4632) -> (0, -73.5)
  line L6 (0, -70.4632) -> (0, -67.4265)
  line L7 (0, -70.4632) -> (18.8061, -70.4632)
  line L8 (9.4031, -70.4632) -> (7.4031, -70.4632)
  line L9 (7.4031, -70.4632) -> (7.4031, -69.1132)
  line L10 (7.4031, -69.1132) -> (11.4031, -69.1132)
  line L11 (11.4031, -69.1132) -> (11.4031, -71.8132)
  line L12 (11.4031, -71.8132) -> (7.4031, -71.8132)
  line L13 (7.4031, -71.8132) -> (7.4031, -70.4632)
  line L14 (-7.4031, -70.4632) -> (-7.4031, -69.1132)
  line L15 (-7.4031, -69.1132) -> (-11.4031, -69.1132)
  line L16 (-11.4031, -69.1132) -> (-11.4031, -71.8132)
  line L17 (-11.4031, -71.8132) -> (-7.4031, -71.8132)
  line L18 (-7.4031, -71.8132) -> (-7.4031, -70.4632)
  arc A0 (-19.5877, 73.4324) -> (-19.5877, -73.4324) centre (0, 0) ccw projected
  line L19 (-76, 0) -> (51, 0)
  line L20 (51, 51.7204) -> (51, -51.7204) projected
  line L21 (7.4031, 70.4632) -> (7.4031, 69.1132)
  line L22 (7.4031, 69.1132) -> (11.4031, 69.1132)
  line L23 (11.4031, 69.1132) -> (11.4031, 71.8132)
  line L24 (11.4031, 71.8132) -> (7.4031, 71.8132)
  line L25 (7.4031, 71.8132) -> (7.4031, 70.4632)
  line L26 (-7.4031, 69.1132) -> (-11.4031, 69.1132)
  line L27 (-11.4031, 69.1132) -> (-11.4031, 71.8132)
  line L28 (-11.4031, 71.8132) -> (-7.4031, 71.8132)
  line L29 (-7.4031, 71.8132) -> (-7.4031, 70.4632)
  line L30 (-7.4031, 70.4632) -> (-7.4031, 69.1132)
  line L31 (11.4031, -70.4632) -> (11.4031, -71.8132)
  line L32 (7.4031, -71.8132) -> (7.4031, -70.4632)
  line L33 (7.4031, -69.1132) -> (7.4031, -70.4632)
  line L34 (7.4031, -69.1132) -> (11.4031, -69.1132)
  line L35 (11.4031, -71.8132) -> (7.4031, -71.8132)
  dimension "d144" = 2
  dimension "d145" = 1.35
  dimension "d146" = 4
  dimension "d147" = 2.7
  dimension "d148" = 4
  constraints: 66 end point, 15 symmetric about line, 8 midpoint, 8 perpendicular, 7 point on line, 2 collinear, 1 point on circle, 1 vertical
  measures "d144" distance of L8.start L8.end
  measures "d145" distance of L8.end L9.end
  measures "d146" distance of L9.end L10.end
  measures "d147" distance of L10.end L11.end
  measures "d148" distance of L11.end L12.end
extrude "Extrusion8" cut sketch "Sketch9" against normal blind 49.25 contours L11 L12 L13 L4 | L4 L9 L10 L11 | L18 L17 L16 L4 | L4 L16 L15 L14 | L25 L24 L23 L22 L21 | L26 L27 L28 L29 L30 bodies 3
body "Solid1"
body "Solid2"
body "Solid3"
